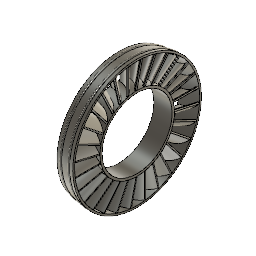
petrol_turbine_three_eng_model (Autodesk Fusion 360 design; units mm, degrees)
Autodesk Fusion 360 part; units mm, degrees
sketch "Sketch1" plane through (0, 0, 0) normal (1, 0, 0) x (0, 1, 0)
  circle A0 centre (0, 0) radius 37.945
  circle A1 centre (0, 0) radius 40.445
  dimension "d1" = 75.89
  dimension "d2" = 80.89
  constraint coincident A0.centre A1.centre
  measures "d1" diameter of A0
  measures "d2" diameter of A1
extrude "Extrude1" add sketch "Sketch1" along normal blind 20 makes body 1
sketch "Sketch2" plane through (0, 0, 0) normal (0, 1, 0) x (1, 0, 0)
  line L0 (0, -40.445) -> (0, 40.445)
  line L1 (20, -40.445) -> (20, 40.445)
  line L2 (0, 0) -> (0, -103.0739) construction
  line L3 (20, 0) -> (20, -103.0739) construction
  line L4 (0, -65.265) -> (20, -67.945)
  line L5 (0, -67.2829) -> (0, -65.265)
  line L6 (20, -69.9629) -> (20, -67.945)
  arc A0 (4.0089, -67.8201) -> (5.9911, -68.0857) centre (5, -67.9529) ccw
  line L7 (0, -67.2829) -> (4.0089, -67.8201)
  arc A1 (14.0089, -69.1601) -> (15.9911, -69.4257) centre (15, -69.2929) ccw
  line L8 (5.9911, -68.0857) -> (14.0089, -69.1601)
  line L9 (15.9911, -69.4257) -> (20, -69.9629)
  dimension "d5" = 67.945
  dimension "d6" = 65.265
  dimension "d7" = 2
  dimension "d8" = 2
  dimension "d9" = 2
  dimension "d10" = 5
  dimension "d11" = 5
  constraint coincident L2.start origin
  constraint parallel L0 L2
  constraint midpoint L1 L3.start
  constraint parallel L1 L3
  constraint coincident L2 L4.start
  constraint coincident L3 L4.end
  constraint coincident L2 L5.start
  constraint coincident L3 L6.start
  constraint parallel L4 L7
  constraint coincident A0.centre L7
  constraint coincident A1.centre L7
  constraint coincident A0.end L7
  constraint collinear L7 L8
  constraint coincident A1.end L8
  constraint collinear L8 L9
  measures "d5" distance of L3.start L4.end
  measures "d6" distance of L2.start L4.start
  measures "d7" distance of L4 L7
  measures "d8" diameter of A0
  measures "d9" diameter of A1
  measures "d10" horizontal distance of L5.start A0.centre
  measures "d11" horizontal distance of L6.start A1.centre
revolve "Revolve1" add sketch "Sketch2" angle 360 about axis through (1.75, 0, 0) along (1, 0, 0) separate body makes body 2
sketch "Sketch3" plane through (0, 0, 0) normal (0, 1, 0) x (1, 0, 0)
  line L0 (0, 67.2829) -> (0, -67.2829)
  line L1 (20, 69.9629) -> (20, -69.9629)
  line L2 (15.9911, -69.4257) -> (20, -69.9629)
  line L3 (15.9911, 69.4257) -> (20, 69.9629)
  arc A0 (14, -69.2929) -> (15.9911, -69.4257) centre (15, -69.2929) ccw
  arc A1 (15.9911, 69.4257) -> (14, 69.2929) centre (15, 69.2929) ccw
  line L4 (14, 69.2929) -> (14, 69.1589)
  line L5 (14, -69.1589) -> (14, -69.2929)
  line L6 (5.9911, -68.0857) -> (14, -69.1589)
  line L7 (5.9911, 68.0857) -> (14, 69.1589)
  arc A2 (4, -67.9529) -> (5.9911, -68.0857) centre (5, -67.9529) ccw
  arc A3 (5.9911, 68.0857) -> (4, 67.9529) centre (5, 67.9529) ccw
  line L8 (4, 67.9529) -> (4, 67.8189)
  line L9 (4, -67.8189) -> (4, -67.9529)
  line L10 (0, -67.2829) -> (4, -67.8189)
  line L11 (0, 67.2829) -> (4, 67.8189)
  line L12 (0, 67.2829) -> (4, 67.8189)
  line L13 (5.9911, 68.0857) -> (14, 69.1589)
  line L14 (15.9911, 69.4257) -> (20, 69.9629)
  line L15 (20, 69.9629) -> (20, 79.9328)
  line L16 (0, 67.2829) -> (0, 79.9328)
  line L17 (20, 79.9328) -> (18.9877, 79.9328)
  line L18 (18.9877, 79.9328) -> (0, 79.9328)
  arc A4 (15.9911, 69.4257) -> (14, 69.2929) centre (15, 69.2929) ccw
  arc A5 (5.9911, 68.0857) -> (4, 67.9529) centre (5, 67.9529) ccw
  constraint coincident L0.start L11.start
  constraint coincident L8.end L11.end
  constraint coincident L7.start A3.start
  constraint coincident L4.end L7.end
  constraint coincident L3.start A1.start
  constraint coincident L1.start L3.end
  constraint parallel L1 L15
  constraint parallel L0 L16
  constraint perpendicular L15 L17
  constraint perpendicular L15 L18
  constraint concentric A3 A5
  constraint concentric A1 A4
sketch "Sketch4" plane through (0, 0, 0) normal (0, 0, 1) x (1, 0, 0)
  line L0 (20, 69.9629) -> (20, -69.9629)
  arc A0 (19.8634, -9.4954) -> (0.9723, 0.9996) centre (1.5599, -20.1922) ccw
  arc A1 (18.1366, -10.5046) -> (1.0277, -0.9996) centre (1.5599, -20.1922) ccw
  line L1 (1.0277, -0.9996) -> (0.9723, 0.9996)
  line L2 (18.1366, -10.5046) -> (19.8634, -9.4954)
  point P0 (1, 0)
  point P1 (19, -10)
  point P2 (20, 0)
  dimension "d13" = 1
  dimension "d14" = 1
  dimension "d15" = 10
  measures "d13" distance of P0 origin
  measures "d14" distance of P1 L0
  measures "d15" vertical distance of P1 P2
extrude "Extrude2" add sketch "Sketch4" along normal blind 69 separate body makes body 3
fillet "Fillet1" radius 1 4 edges at (19.8634, -9.4954, 34.5) (18.1366, -10.5046, 34.5) (1.0277, -0.9996, 34.5) (0.9723, 0.9996, 34.5) on bodies 3
pattern_circular "C-Pattern1" count 28 over 360 about axis through (1.75, 0, 0) along (1, 0, 0) of "Extrude2", "Fillet1" makes body 4 at (8.7363, -5.3557, 22.3691) makes body 5 at (18.1658, -26.2775, 38.4016) makes body 6 at (13.9234, -31.0031, 34.1121) makes body 7 at (9.6503, -36.3363, 28.214) makes body 8 at (13.9234, -42.7335, 17.2822) makes body 9 at (8.7363, -22.4776, 4.8803) makes body 10 at (18.1658, -46, -7.0134) makes body 11 at (9.6503, -44.7139, -10.8177) makes body 12 at (8.7363, -20.6165, -10.199) makes body 13 at (16.185, -32.9436, -32.4683) makes body 14 at (9.6503, -28.214, -36.3363) makes body 15 at (18.1658, -13.6398, -44.4875) makes body 16 at (8.7363, -4.8803, -22.4776) makes body 17 at (9.6503, 0.5967, -46) makes body 18 at (9.6503, 10.8177, -44.7139) makes body 19 at (9.6503, 20.4963, -41.1857) makes body 20 at (13.9234, 31.0031, -34.1121) makes body 21 at (13.9234, 37.8164, -26.358) makes body 22 at (16.185, 43.5466, -15.5937) makes body 23 at (8.7363, 44.9009, -9.9982) makes body 24 at (9.6503, 46, 0.5967) makes body 25 at (13.9234, 44.1857, 13.1321) makes body 26 at (13.9234, 40.1557, 22.6351) makes body 27 at (8.7363, 35.8122, 28.8712) makes body 28 at (9.6503, 28.214, 36.3363) makes body 29 at (9.6503, 19.421, 41.7035) makes body 30 at (8.7363, 4.8803, 22.4776)
revolve "Revolve2" cut sketch "Sketch3" angle 360 about axis through (1.75, 0, 0) along (1, 0, 0) contours L3 A1 L4 L7 A3 L8 L11 L12 L13 L14 L15 L16 L17 L18 A4 A5 bodies 3 4 5 6 7 8 9 10 11 12 13 14 15 16 17 18 19 20 21 22 23 24 25 26 27 28 29 30
sketch "Sketch5" plane through (20, 0, 0) normal (1, 0, 0) x (0, 1, 0)
  circle A0 centre (0, 0) radius 37.945
  circle A1 centre (0, 0) radius 40.445
  circle A2 centre (0, 0) radius 37.945
  dimension "d26" = 75.89
  constraint coincident A0.centre A1.centre
  measures "d26" diameter of A2
extrude "Extrude3" cut sketch "Sketch5" against normal blind 25 contours A0 A2 bodies 3 4 5 6 7 8 9 10 11 12 13 14 15 16 17 18 19 20 21 22 23 24 25 26 27 28 29 30
combine "Combine1" operation add target body 2 tool bodies 8 23 24 6 30 3 4 5 21 11 1 10 18 17 16 20 13 15 22 9 12 14 19 27 28 26 29 7 25
equation "d5 = ( 135.89 / 2 ) * 1 mm"
equation "d6 = ( 130.53 / 2 ) * 1 mm"
equation "d19 = ( 138 / 2 ) * 1 mm"
